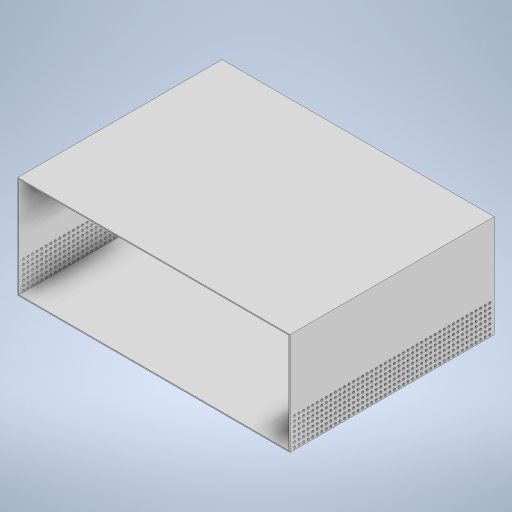
# Autodesk Inventor part: Dustbin Body
Saved by Autodesk Inventor 2024 (Build 280153000, 153)
## iProperties
Created: 2024-09-03
Part Number: Dustbin Body
Material: Generic
Document SubType Name: Modeling
Designer: srira
Density: 1 g/cm^3
Appearance: Default
Author: srira
Autodesk Inventor part; units mm, degrees
ref_plane "YZ Plane" through (0, 0, 0) normal (1, 0, 0) x (0, 1, 0)
ref_plane "XZ Plane" through (0, 0, 0) normal (0, 1, 0) x (-1, 0, 0)
ref_plane "XY Plane" through (0, 0, 0) normal (0, 0, 1) x (1, 0, 0)
sketch "Sketch1" plane through (0, 0, 0) normal (0, 0, 1) x (1, 0, 0)
  line L0 (-312.0409, 305.3441) -> (887.9591, 305.3441)
  line L1 (887.9591, 305.3441) -> (887.9591, -144.6559)
  line L2 (887.9591, -144.6559) -> (-312.0409, -144.6559)
  line L3 (-312.0409, -144.6559) -> (-312.0409, 305.3441)
  point P0 (0, 0)
  dimension "d0" = 1200
  dimension "d1" = 450
  constraints: 8 end point, 2 parallel, 1 horizontal, 1 perpendicular
  measures "d0" distance of L1.end L2.end
  measures "d1" distance of L0.end L1.end
extrude "Extrusion1" add sketch "Sketch1" along normal blind 900
sketch "Sketch2" plane through (0, 0, 900) normal (0, 0, 1) x (1, 0, 0)
  line L0 (-307.0409, 300.344) -> (882.9591, 300.344)
  line L1 (882.9591, 300.344) -> (882.9591, -139.656)
  line L2 (882.9591, -139.656) -> (-307.0409, -139.656)
  line L3 (-307.0409, -139.656) -> (-307.0409, 300.344)
  line L4 (-307.0409, 300.344) -> (882.9591, -139.656) construction
  line L5 (882.9591, 300.344) -> (-307.0409, -139.656) construction
  point P0 (0, 0)
  point P1 (287.9591, 80.344)
  dimension "d4" = 1190
  dimension "d5" = 440
  constraints: 12 end point, 2 midpoint, 2 parallel, 1 horizontal, 1 perpendicular
  measures "d4" distance of L1.end L2.end
  measures "d5" distance of L0.end L1.end
extrude "Extrusion2" cut sketch "Sketch2" against normal blind 895
sketch "Sketch3" plane through (-312.0409, -144.6559, 0) normal (-1, 0, 0) x (0, 0, 1)
  circle A0 centre (20, 130) radius 5
  line L0 (0, 450) -> (900, 450) projected
  line L1 (33.7696, 450) -> (130.2583, 450)
  point P0 (0, 144.6559)
  dimension "d8" = 10
  constraints: 2 end point, 2 point on line, 1 centre point
  measures "d8" diameter of A0
extrude "Extrusion3" cut sketch "Sketch3" against normal blind 1200
sketch "Sketch4" plane through (-312.0409, -144.6559, 0) normal (-1, 0, 0) x (0, 0, 1)
  circle A0 centre (20, 130) radius 5 projected
  circle A1 centre (20, 130) radius 5
  line L0 (0, 450) -> (900, 450) projected
  line L1 (32.7704, 450) -> (108.1312, 450)
  line L2 (0, 89.5845) -> (0, 22.0197)
  line L3 (0, 0) -> (0, 450) projected
  circle A2 centre (40, 130) radius 5
  circle A3 centre (60, 130) radius 5
  circle A4 centre (80, 130) radius 5
  circle A5 centre (100, 130) radius 5
  circle A6 centre (120, 130) radius 5
  circle A7 centre (140, 130) radius 5
  circle A8 centre (160, 130) radius 5
  circle A9 centre (180, 130) radius 5
  circle A10 centre (200, 130) radius 5
  circle A11 centre (220, 130) radius 5
  circle A12 centre (240, 130) radius 5
  circle A13 centre (260, 130) radius 5
  circle A14 centre (280, 130) radius 5
  circle A15 centre (300, 130) radius 5
  circle A16 centre (320, 130) radius 5
  circle A17 centre (340, 130) radius 5
  circle A18 centre (360, 130) radius 5
  circle A19 centre (380, 130) radius 5
  circle A20 centre (400, 130) radius 5
  circle A21 centre (420, 130) radius 5
  circle A22 centre (440, 130) radius 5
  circle A23 centre (460, 130) radius 5
  circle A24 centre (480, 130) radius 5
  circle A25 centre (500, 130) radius 5
  circle A26 centre (520, 130) radius 5
  circle A27 centre (540, 130) radius 5
  circle A28 centre (560, 130) radius 5
  circle A29 centre (580, 130) radius 5
  circle A30 centre (600, 130) radius 5
  circle A31 centre (620, 130) radius 5
  circle A32 centre (640, 130) radius 5
  circle A33 centre (660, 130) radius 5
  circle A34 centre (680, 130) radius 5
  circle A35 centre (700, 130) radius 5
  circle A36 centre (720, 130) radius 5
  circle A37 centre (740, 130) radius 5
  circle A38 centre (760, 130) radius 5
  circle A39 centre (780, 130) radius 5
  circle A40 centre (800, 130) radius 5
  circle A41 centre (820, 130) radius 5
  circle A42 centre (840, 130) radius 5
  circle A43 centre (860, 130) radius 5
  circle A44 centre (880, 130) radius 5
  circle A45 centre (20, 110) radius 5
  circle A46 centre (40, 110) radius 5
  circle A47 centre (60, 110) radius 5
  circle A48 centre (80, 110) radius 5
  circle A49 centre (100, 110) radius 5
  circle A50 centre (120, 110) radius 5
  circle A51 centre (140, 110) radius 5
  circle A52 centre (160, 110) radius 5
  circle A53 centre (180, 110) radius 5
  circle A54 centre (200, 110) radius 5
  circle A55 centre (220, 110) radius 5
  circle A56 centre (240, 110) radius 5
  circle A57 centre (260, 110) radius 5
  circle A58 centre (280, 110) radius 5
  circle A59 centre (300, 110) radius 5
  circle A60 centre (320, 110) radius 5
  circle A61 centre (340, 110) radius 5
  circle A62 centre (360, 110) radius 5
  circle A63 centre (380, 110) radius 5
  circle A64 centre (400, 110) radius 5
  circle A65 centre (420, 110) radius 5
  circle A66 centre (440, 110) radius 5
  circle A67 centre (460, 110) radius 5
  circle A68 centre (480, 110) radius 5
  circle A69 centre (500, 110) radius 5
  circle A70 centre (520, 110) radius 5
  circle A71 centre (540, 110) radius 5
  circle A72 centre (560, 110) radius 5
  circle A73 centre (580, 110) radius 5
  circle A74 centre (600, 110) radius 5
  circle A75 centre (620, 110) radius 5
  circle A76 centre (640, 110) radius 5
  circle A77 centre (660, 110) radius 5
  circle A78 centre (680, 110) radius 5
  circle A79 centre (700, 110) radius 5
  circle A80 centre (720, 110) radius 5
  circle A81 centre (740, 110) radius 5
  circle A82 centre (760, 110) radius 5
  circle A83 centre (780, 110) radius 5
  circle A84 centre (800, 110) radius 5
  circle A85 centre (820, 110) radius 5
  circle A86 centre (840, 110) radius 5
  circle A87 centre (860, 110) radius 5
  circle A88 centre (880, 110) radius 5
  circle A89 centre (20, 90) radius 5
  circle A90 centre (40, 90) radius 5
  circle A91 centre (60, 90) radius 5
  circle A92 centre (80, 90) radius 5
  circle A93 centre (100, 90) radius 5
  circle A94 centre (120, 90) radius 5
  circle A95 centre (140, 90) radius 5
  circle A96 centre (160, 90) radius 5
  circle A97 centre (180, 90) radius 5
  circle A98 centre (200, 90) radius 5
  circle A99 centre (220, 90) radius 5
  circle A100 centre (240, 90) radius 5
  circle A101 centre (260, 90) radius 5
  circle A102 centre (280, 90) radius 5
  circle A103 centre (300, 90) radius 5
  circle A104 centre (320, 90) radius 5
  circle A105 centre (340, 90) radius 5
  circle A106 centre (360, 90) radius 5
  circle A107 centre (380, 90) radius 5
  circle A108 centre (400, 90) radius 5
  circle A109 centre (420, 90) radius 5
  circle A110 centre (440, 90) radius 5
  circle A111 centre (460, 90) radius 5
  circle A112 centre (480, 90) radius 5
  circle A113 centre (500, 90) radius 5
  circle A114 centre (520, 90) radius 5
  circle A115 centre (540, 90) radius 5
  circle A116 centre (560, 90) radius 5
  circle A117 centre (580, 90) radius 5
  circle A118 centre (600, 90) radius 5
  circle A119 centre (620, 90) radius 5
  circle A120 centre (640, 90) radius 5
  circle A121 centre (660, 90) radius 5
  circle A122 centre (680, 90) radius 5
  circle A123 centre (700, 90) radius 5
  circle A124 centre (720, 90) radius 5
  circle A125 centre (740, 90) radius 5
  circle A126 centre (760, 90) radius 5
  circle A127 centre (780, 90) radius 5
  circle A128 centre (800, 90) radius 5
  circle A129 centre (820, 90) radius 5
  circle A130 centre (840, 90) radius 5
  circle A131 centre (860, 90) radius 5
  circle A132 centre (880, 90) radius 5
  circle A133 centre (20, 70) radius 5
  circle A134 centre (40, 70) radius 5
  circle A135 centre (60, 70) radius 5
  circle A136 centre (80, 70) radius 5
  circle A137 centre (100, 70) radius 5
  circle A138 centre (120, 70) radius 5
  circle A139 centre (140, 70) radius 5
  circle A140 centre (160, 70) radius 5
  circle A141 centre (180, 70) radius 5
  circle A142 centre (200, 70) radius 5
  circle A143 centre (220, 70) radius 5
  circle A144 centre (240, 70) radius 5
  circle A145 centre (260, 70) radius 5
  circle A146 centre (280, 70) radius 5
  circle A147 centre (300, 70) radius 5
  circle A148 centre (320, 70) radius 5
  circle A149 centre (340, 70) radius 5
  circle A150 centre (360, 70) radius 5
  circle A151 centre (380, 70) radius 5
  circle A152 centre (400, 70) radius 5
  circle A153 centre (420, 70) radius 5
  circle A154 centre (440, 70) radius 5
  circle A155 centre (460, 70) radius 5
  circle A156 centre (480, 70) radius 5
  circle A157 centre (500, 70) radius 5
  circle A158 centre (520, 70) radius 5
  circle A159 centre (540, 70) radius 5
  circle A160 centre (560, 70) radius 5
  circle A161 centre (580, 70) radius 5
  circle A162 centre (600, 70) radius 5
  circle A163 centre (620, 70) radius 5
  circle A164 centre (640, 70) radius 5
  circle A165 centre (660, 70) radius 5
  circle A166 centre (680, 70) radius 5
  circle A167 centre (700, 70) radius 5
  circle A168 centre (720, 70) radius 5
  circle A169 centre (740, 70) radius 5
  circle A170 centre (760, 70) radius 5
  circle A171 centre (780, 70) radius 5
  circle A172 centre (800, 70) radius 5
  circle A173 centre (820, 70) radius 5
  circle A174 centre (840, 70) radius 5
  circle A175 centre (860, 70) radius 5
  circle A176 centre (880, 70) radius 5
  circle A177 centre (20, 50) radius 5
  circle A178 centre (40, 50) radius 5
  circle A179 centre (60, 50) radius 5
  circle A180 centre (80, 50) radius 5
  circle A181 centre (100, 50) radius 5
  circle A182 centre (120, 50) radius 5
  circle A183 centre (140, 50) radius 5
  circle A184 centre (160, 50) radius 5
  circle A185 centre (180, 50) radius 5
  circle A186 centre (200, 50) radius 5
  circle A187 centre (220, 50) radius 5
  circle A188 centre (240, 50) radius 5
  circle A189 centre (260, 50) radius 5
  circle A190 centre (280, 50) radius 5
  circle A191 centre (300, 50) radius 5
  circle A192 centre (320, 50) radius 5
  circle A193 centre (340, 50) radius 5
  circle A194 centre (360, 50) radius 5
  circle A195 centre (380, 50) radius 5
  circle A196 centre (400, 50) radius 5
  circle A197 centre (420, 50) radius 5
  circle A198 centre (440, 50) radius 5
  circle A199 centre (460, 50) radius 5
  circle A200 centre (480, 50) radius 5
  circle A201 centre (500, 50) radius 5
  circle A202 centre (520, 50) radius 5
  circle A203 centre (540, 50) radius 5
  circle A204 centre (560, 50) radius 5
  circle A205 centre (580, 50) radius 5
  circle A206 centre (600, 50) radius 5
  circle A207 centre (620, 50) radius 5
  circle A208 centre (640, 50) radius 5
  circle A209 centre (660, 50) radius 5
  circle A210 centre (680, 50) radius 5
  circle A211 centre (700, 50) radius 5
  circle A212 centre (720, 50) radius 5
  circle A213 centre (740, 50) radius 5
  circle A214 centre (760, 50) radius 5
  circle A215 centre (780, 50) radius 5
  circle A216 centre (800, 50) radius 5
  circle A217 centre (820, 50) radius 5
  circle A218 centre (840, 50) radius 5
  circle A219 centre (860, 50) radius 5
  circle A220 centre (880, 50) radius 5
  circle A221 centre (20, 30) radius 5
  circle A222 centre (40, 30) radius 5
  circle A223 centre (60, 30) radius 5
  circle A224 centre (80, 30) radius 5
  circle A225 centre (100, 30) radius 5
  circle A226 centre (120, 30) radius 5
  circle A227 centre (140, 30) radius 5
  circle A228 centre (160, 30) radius 5
  circle A229 centre (180, 30) radius 5
  circle A230 centre (200, 30) radius 5
  circle A231 centre (220, 30) radius 5
  circle A232 centre (240, 30) radius 5
  circle A233 centre (260, 30) radius 5
  circle A234 centre (280, 30) radius 5
  circle A235 centre (300, 30) radius 5
  circle A236 centre (320, 30) radius 5
  circle A237 centre (340, 30) radius 5
  circle A238 centre (360, 30) radius 5
  circle A239 centre (380, 30) radius 5
  circle A240 centre (400, 30) radius 5
  circle A241 centre (420, 30) radius 5
  circle A242 centre (440, 30) radius 5
  circle A243 centre (460, 30) radius 5
  circle A244 centre (480, 30) radius 5
  circle A245 centre (500, 30) radius 5
  circle A246 centre (520, 30) radius 5
  circle A247 centre (540, 30) radius 5
  circle A248 centre (560, 30) radius 5
  circle A249 centre (580, 30) radius 5
  circle A250 centre (600, 30) radius 5
  circle A251 centre (620, 30) radius 5
  circle A252 centre (640, 30) radius 5
  circle A253 centre (660, 30) radius 5
  circle A254 centre (680, 30) radius 5
  circle A255 centre (700, 30) radius 5
  circle A256 centre (720, 30) radius 5
  circle A257 centre (740, 30) radius 5
  circle A258 centre (760, 30) radius 5
  circle A259 centre (780, 30) radius 5
  circle A260 centre (800, 30) radius 5
  circle A261 centre (820, 30) radius 5
  circle A262 centre (840, 30) radius 5
  circle A263 centre (860, 30) radius 5
  circle A264 centre (880, 30) radius 5
  circle A265 centre (20, 10) radius 5
  circle A266 centre (40, 10) radius 5
  circle A267 centre (60, 10) radius 5
  circle A268 centre (80, 10) radius 5
  circle A269 centre (100, 10) radius 5
  circle A270 centre (120, 10) radius 5
  circle A271 centre (140, 10) radius 5
  circle A272 centre (160, 10) radius 5
  circle A273 centre (180, 10) radius 5
  circle A274 centre (200, 10) radius 5
  circle A275 centre (220, 10) radius 5
  circle A276 centre (240, 10) radius 5
  circle A277 centre (260, 10) radius 5
  circle A278 centre (280, 10) radius 5
  circle A279 centre (300, 10) radius 5
  circle A280 centre (320, 10) radius 5
  circle A281 centre (340, 10) radius 5
  circle A282 centre (360, 10) radius 5
  circle A283 centre (380, 10) radius 5
  circle A284 centre (400, 10) radius 5
  circle A285 centre (420, 10) radius 5
  circle A286 centre (440, 10) radius 5
  circle A287 centre (460, 10) radius 5
  circle A288 centre (480, 10) radius 5
  circle A289 centre (500, 10) radius 5
  circle A290 centre (520, 10) radius 5
  circle A291 centre (540, 10) radius 5
  circle A292 centre (560, 10) radius 5
  circle A293 centre (580, 10) radius 5
  circle A294 centre (600, 10) radius 5
  circle A295 centre (620, 10) radius 5
  circle A296 centre (640, 10) radius 5
  circle A297 centre (660, 10) radius 5
  circle A298 centre (680, 10) radius 5
  circle A299 centre (700, 10) radius 5
  circle A300 centre (720, 10) radius 5
  circle A301 centre (740, 10) radius 5
  circle A302 centre (760, 10) radius 5
  circle A303 centre (780, 10) radius 5
  circle A304 centre (800, 10) radius 5
  circle A305 centre (820, 10) radius 5
  circle A306 centre (840, 10) radius 5
  circle A307 centre (860, 10) radius 5
  circle A308 centre (880, 10) radius 5
  point P0 (0, 144.6559)
  dimension "d11" = 10
  dimension "d14" = 20
  dimension "d17" = 20
  constraints: 308 centre point, 4 end point, 3 point on line, 1 coincident, 1 horizontal, 1 vertical, 614 other
  measures "d11" diameter of A1
  measures "d14" distance of A1.centre A2.centre
  measures "d17" distance of A1.centre A45.centre
extrude "Extrusion4" cut sketch "Sketch4" against normal blind 1200 contours A2 | A3 | A4 | A5 | A6 | A7 | A8 | A9 | A10 | A11 | A12 | A13 | A14 | A15 | A16 | A17 | A18 | A19 | A20 | A21 | A22 | A23 | A24 | A25 | A26 | A27 | A28 | A29 | A30 | A31 | A32 | A33 | A34 | A35 | A36 | A37 | A38 | A39 | A40 | A41 | A42 | A43 | A44 | A45 | A46 | A47 | A48 | A49 | A50 | A51 | A52 | A53 | A54 | A55 | A56 | A57 | A58 | A59 | A60 | A61 | A62 | A63 | A64 | A65 | A66 | A67 | A68 | A69 | A70 | A71 | A72 | A73 | A74 | A75 | A76 | A77 | A78 | A79 | A80 | A81 | A82 | A83 | A84 | A85 | A86 | A87 | A88 | A89 | A90 | A91 | A92 | A93 | A94 | A95 | A96 | A97 | A98 | A99 | A100 | A101 | A102 | A103 | A104 | A105 | A106 | A107 | A108 | A109 | A110 | A111 | A112 | A113 | A114 | A115 | A116 | A117 | A118 | A119 | A120 | A121 | A122 | A123 | A124 | A125 | A126 | A127 | A128 | A129 | A130 | A131 | A132 | A133 | A134 | A135 | A136 | A137 | A138 | A139 | A140 | A141 | A142 | A143 | A144 | A145 | A146 | A147 | A148 | A149 | A150 | A151 | A152 | A153 | A154 | A155 | A156 | A157 | A158 | A159 | A160 | A161 | A162 | A163 | A164 | A165 | A166 | A167 | A168 | A169 | A170 | A171 | A172 | A173 | A174 | A175 | A176 | A177 | A178 | A179 | A180 | A181 | A182 | A183 | A184 | A185 | A186 | A187 | A188 | A189 | A190 | A191 | A192 | A193 | A194 | A195 | A196 | A197 | A198 | A199 | A200 | A201 | A202 | A203 | A204 | A205 | A206 | A207 | A208 | A209 | A210 | A211 | A212 | A213 | A214 | A215 | A216 | A217 | A218 | A219 | A220 | A221 | A222 | A223 | A224 | A225 | A226 | A227 | A228 | A229 | A230 | A231 | A232 | A233 | A234 | A235 | A236 | A237 | A238 | A239 | A240 | A241 | A242 | A243 | A244 | A245 | A246 | A247 | A248 | A249 | A250 | A251 | A252 | A253 | A254 | A255 | A256 | A257 | A258 | A259 | A260 | A261 | A262 | A263 | A264 | A265 | A266 | A267 | A268 | A269 | A270 | A271 | A272 | A273 | A274 | A275 | A276 | A277 | A278 | A279 | A280 | A281 | A282 | A283 | A284 | A285 | A286 | A287 | A288 | A289 | A290 | A291 | A292 | A293 | A294 | A295 | A296 | A297 | A298 | A299 | A300 | A301 | A302 | A303 | A304 | A305 | A306 | A307 | A308
body "Solid1"
